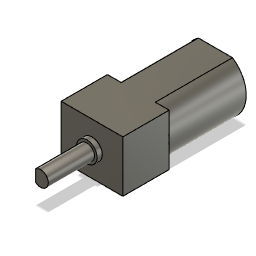
Motor' v1 (Autodesk Fusion 360 design; units mm, degrees)
Autodesk Fusion 360 part; units mm, degrees
note: some values were not read from the file. Set by a fixed rule: which sketch regions a step uses.
sketch "Sketch1" plane through (0, 0, 0) normal (0, 0, 1) x (1, 0, 0)
  line L0 (-5, 5) -> (5, 5)
  line L1 (5, 5) -> (5, -5)
  line L2 (5, -5) -> (-5, -5)
  line L3 (-5, -5) -> (-5, 5)
  line L4 (-5, 5) -> (5, -5) construction
  line L5 (5, 5) -> (-5, -5) construction
  circle A0 centre (0, 0) radius 6
  dimension "d1" = 10
  dimension "d2" = 10
  dimension "d3" = 12
  constraint horizontal L0
  constraint perpendicular L0 L1
  constraint parallel L0 L2
  constraint parallel L1 L3
  constraint coincident L4 A0.centre
  constraint coincident L5 A0.centre
  constraint coincident A0.centre origin
  measures "d1" distance of L1.end L2.end
  measures "d2" distance of L0.end L1.end
  measures "d3" diameter of A0
extrude "Extrude1" add sketch "Sketch1" along normal blind 15 contours L0 L1 L2 L3 A0 | L3 A0 | L1 A0 makes body 1
sketch "Sketch2" plane through (0, 0, 15) normal (0, 0, 1) x (1, 0, 0)
  arc A0 (-3.3166, 5) -> (-3.3166, -5) centre (0, 0) ccw
  line L0 (-3.3166, -5) -> (3.3166, -5)
  arc A1 (3.3166, -5) -> (3.3166, 5) centre (0, 0) ccw
  line L1 (3.3166, 5) -> (-3.3166, 5)
  line L2 (-6, 5) -> (6, 5)
  line L3 (6, 5) -> (6, -5)
  line L4 (6, -5) -> (-6, -5)
  line L5 (-6, -5) -> (-6, 5)
  line L6 (-6, 5) -> (6, -5) construction
  line L7 (6, 5) -> (-6, -5) construction
  dimension "d6" = 10
  constraint horizontal L2
  constraint perpendicular L2 L3
  constraint parallel L2 L4
  constraint parallel L3 L5
  constraint coincident L6 A0.centre
  constraint coincident L7 A0.centre
  constraint coincident A0.centre A1.centre
  measures "d6" distance of L2.end L3.end
extrude "Extrude2" add sketch "Sketch2" along normal blind 9 bodies 1
sketch "Sketch3" plane through (0, 0, 24) normal (0, 0, 1) x (1, 0, 0)
  line L0 (-6, -5) -> (6, -5)
  line L1 (6, -5) -> (6, 5)
  line L2 (6, 5) -> (-6, 5)
  line L3 (-6, 5) -> (-6, -5)
  circle A0 centre (0, 0) radius 1.5
  line L4 (0, 2) -> (0, -2) construction
  line L5 (0, 0) -> (1.5, 0) construction
  line L6 (1.5, 0) -> (-0.97, 0) construction
  line L7 (-2.5, 2) -> (-0.97, 2)
  line L8 (-0.97, 2) -> (-0.97, -1.75)
  line L9 (-0.97, -1.75) -> (-2.5, -1.75)
  line L10 (-2.5, -1.75) -> (-2.5, 2)
  dimension "d9" = 3
  dimension "d10" = 2.47
  constraint coincident A0.centre L5.start
  constraint vertical L4
  constraint coincident A0 L5.end
  constraint perpendicular L4 L5
  constraint perpendicular L4 L6
  constraint horizontal L7
  constraint vertical L8
  constraint horizontal L9
  constraint vertical L10
  measures "d9" diameter of A0
  measures "d10" distance of L5.end L6.end
extrude "Extrude3" add sketch "Sketch3" along normal blind 10 contours A0 L8 picked at (-0.2031, 0.3765) bodies 1
sketch "Sketch4" plane through (0, 0, 24) normal (0, 0, 1) x (1, 0, 0)
  line L0 (-0.97, -1.1442) -> (-0.97, 1.1442)
  arc A0 (-0.97, -1.1442) -> (-0.97, 1.1442) centre (0, 0) ccw
  line L1 (-6, -5) -> (6, -5)
  line L2 (6, -5) -> (6, 5)
  line L3 (6, 5) -> (-6, 5)
  line L4 (-6, 5) -> (-6, -5)
  circle A1 centre (0, 0) radius 2
  dimension "d13" = 4
  constraint concentric A0 A1
  measures "d13" diameter of A1
extrude "Extrude4" add sketch "Sketch4" along normal blind 1 contours A1 bodies 1
copy_body "Body->Comp1" bodies 1 removing the originals makes body 2 in component "Motor"
component "Motor" placed x (1, 0, 0) y (0, 1, 0) z (0, 0, 1) at (0, 0, 0)
